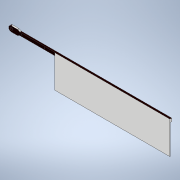
# Autodesk Inventor part: wachlarz_1
Saved by Autodesk Inventor 2022 (Build 260153000, 153)
## iProperties
Created: 2022-12-26
Part Number: wachlarz_1
Material: Generic
Document SubType Name: Modeling
Designer: Kamil
Density: 1 g/cm^3
Appearance: Default
Author: Kamil
Autodesk Inventor part; units mm, degrees
ref_plane "YZ Plane" through (0, 0, 0) normal (1, 0, 0) x (0, 1, 0)
ref_plane "XZ Plane" through (0, 0, 0) normal (0, 1, 0) x (-1, 0, 0)
ref_plane "XY Plane" through (0, 0, 0) normal (0, 0, 1) x (1, 0, 0)
sketch "Sketch1" plane through (0, 0, 0) normal (0, 0, 1) x (1, 0, 0)
  circle A0 centre (0, 3.75) radius 1.75 projected
  line L0 (3.5, -3.25) -> (11.1738, -3.25) projected
  line L1 (11.1738, -3.25) -> (11.1738, -5.25) projected
  line L2 (11.1738, -5.25) -> (-11.1738, -5.25) projected
  line L3 (-11.1738, -5.25) -> (-11.1738, -3.25) projected
  line L4 (-11.1738, -3.25) -> (-3.5, -3.25) projected
  line L5 (-3.5, -3.25) -> (-3.5, 3.75) projected
  arc A1 (3.5, 3.75) -> (-3.5, 3.75) centre (0, 3.75) ccw projected
  line L6 (3.5, 3.75) -> (3.5, -3.25) projected
  line L7 (44, 1.75) -> (50, 1.75) projected
  circle A2 centre (0, 3.75) radius 3.5
  line L8 (0, 3.75) -> (250, 3.75)
  line L9 (50, 1.75) -> (0, 1.75)
  line L10 (0, 1.75) -> (0, 3.75)
  line L11 (0, 3.75) -> (50, 3.75)
  line L12 (50, 3.75) -> (50, 1.75)
  line L13 (50, 1.75) -> (250, 1.75)
  line L14 (250, 1.75) -> (250, 3.75)
  line L15 (250, 3.75) -> (50, 3.75)
  line L16 (50, 3.75) -> (50, 1.75)
  line L17 (0, 1.75) -> (250, 1.75)
  line L18 (250, 1.75) -> (250, 5.75)
  line L19 (250, 5.75) -> (0, 5.75)
  line L20 (0, 5.75) -> (0, 1.75)
  circle A3 centre (0, 3.75) radius 3.5
  point P0 (0, 0)
  point P1 (2.8723, 1.75)
  point P2 (2.8723, 5.75)
  dimension "d0" = 250
  dimension "d1" = 2
  constraints: 26 end point, 6 parallel, 4 horizontal, 3 perpendicular, 2 centre point, 2 coincident, 2 concentric, 1 point on line
  measures "d0" distance of L8.start L8.end
  measures "d1" distance between parallel lines of L8 L19
extrude "Extrusion1" add sketch "Sketch1" along normal blind 2 contours L8 A2 L9 L10 A0 | A0 L20 L19 A1 L8 | A0 L10 L9 A2 A1 L19 L20 | L8 L12 L7 L9 L6 | L6 L9 A2 | A1 L19 L18 L8 | L8 L14 L13 L12
sketch "Sketch2" plane through (0, 0, 2) normal (0, 0, 1) x (1, 0, 0)
  line L0 (13, -15.35) -> (13, -12.35) projected
  line L1 (13, -12.35) -> (14.6, -12.35) projected
  line L2 (14.6, -12.35) -> (14.6, -15.35) projected
  line L3 (14.6, -15.35) -> (13, -15.35) projected
  line L4 (15, -16.35) -> (12.5, -16.35) projected
  line L5 (15, -8.75) -> (15, -16.35) projected
  line L6 (15, -8.75) -> (15, -5.25) projected
  line L7 (12.5, -5.25) -> (15, -5.25) projected
  line L8 (12.5, -16.35) -> (12.5, -5.25) projected
  line L9 (44, -8.25) -> (41.5181, -8.25) projected
  line L10 (44, -9.25) -> (46.5, -9.25) projected
  line L11 (13.75, -5.25) -> (13.75, 7.3756)
  line L12 (44, -8.25) -> (44, 8.5683)
  line L13 (2.8723, 1.75) -> (250, 1.75) projected
  line L14 (250, 1.75) -> (250, 5.75) projected
  line L15 (250, 5.75) -> (2.8723, 5.75) projected
  arc A0 (2.8723, 5.75) -> (2.8723, 1.75) centre (0, 3.75) ccw projected
  circle A1 centre (0, 3.75) radius 1.75 projected
  line L16 (250, 5.75) -> (2.8723, 5.75) projected
  line L17 (13.75, 5.75) -> (13.75, 1.75)
  circle A2 centre (13.75, 3.75) radius 0.5
  line L18 (44, 5.75) -> (44, 1.75)
  line L19 (2.8723, 1.75) -> (250, 1.75) projected
  circle A3 centre (44, 3.75) radius 0.5
  point P0 (0, 0)
  dimension "d4" = 1
  dimension "d5" = 1
  constraints: 8 end point, 8 point on line, 3 midpoint, 2 centre point, 2 vertical
  measures "d4" diameter of A2
  measures "d5" diameter of A3
extrude "Extrusion2" cut sketch "Sketch2" against normal blind 2 contours A2 L11 | L11 A2 | A3 L12 | L12 A3
sketch "Sketch3" plane through (0, 0, 2) normal (0, 0, 1) x (1, 0, 0)
  line L0 (50, -24.1664) -> (50, 13.5237) projected
  circle A0 centre (44, 3.75) radius 0.5 projected
  circle A1 centre (13.75, 3.75) radius 0.5 projected
  line L1 (2.8723, 1.75) -> (250, 1.75) projected
  line L2 (250, 1.75) -> (250, 5.75) projected
  line L3 (250, 5.75) -> (2.8723, 5.75) projected
  arc A2 (2.8723, 5.75) -> (2.8723, 1.75) centre (0, 3.75) ccw projected
  circle A3 centre (0, 3.75) radius 1.75 projected
  line L4 (-50, -43.45) -> (50, -43.45) projected
  line L5 (250, 5.75) -> (57.9443, 5.75)
  line L6 (57.9443, 5.75) -> (57.9443, -37.1171)
  line L7 (57.9443, -37.1171) -> (250, -37.1171)
  line L8 (250, -37.1171) -> (250, 5.75)
  point P0 (0, 0)
  point P1 (57.9443, 5.75)
  constraints: 8 end point, 2 parallel, 1 horizontal, 1 perpendicular
extrude "Extrusion3" add sketch "Sketch3" along normal blind 0.5 contours L6 L3 L2 L1 | L1 L8 L7 L6
sketch "Sketch4" plane through (0, 0, 2.5) normal (0, 0, 1) x (1, 0, 0)
  line L0 (250, -37.1171) -> (250, 5.75) projected
  line L1 (250, 5.75) -> (57.9443, 5.75) projected
  line L2 (57.9443, 5.75) -> (57.9443, -37.1171) projected
  line L3 (57.9443, -37.1171) -> (250, -37.1171) projected
  line L4 (250, -37.1171) -> (250, 1.75) projected
  line L5 (250, -37.1171) -> (210, -37.1171)
  line L6 (210, -37.1171) -> (210, 5.75)
  line L7 (210, 5.75) -> (250, 5.75)
  line L8 (250, 5.75) -> (250, -37.1171)
  point P0 (0, 0)
  dimension "d10" = 40
  constraints: 8 end point, 2 parallel, 1 horizontal, 1 perpendicular, 1 point on line
  measures "d10" distance of L6.end L7.end
extrude "Extrusion4" cut sketch "Sketch4" against normal through all contours L3 L6 L1 L0
sketch "Sketch5" plane through (0, 0, 2) normal (0, 0, 1) x (1, 0, 0)
  line L0 (57.9443, 1.75) -> (57.9443, 5.75) projected
  line L1 (57.9443, 5.75) -> (2.8723, 5.75) projected
  arc A0 (2.8723, 5.75) -> (2.8723, 1.75) centre (0, 3.75) ccw projected
  line L2 (2.8723, 1.75) -> (57.9443, 1.75) projected
  circle A1 centre (44, 3.75) radius 0.5 projected
  circle A2 centre (13.75, 3.75) radius 0.5 projected
  circle A3 centre (0, 3.75) radius 1.75 projected
  arc A4 (2.8723, 5.75) -> (2.8723, 1.75) centre (0, 3.75) ccw projected
  line L3 (0, 0.25) -> (7.7599, 0.25)
  line L4 (8.6265, 0.4475) -> (11.3354, 1.75)
  line L5 (2.8723, 1.75) -> (57.9443, 1.75) projected
  arc A5 (7.7599, 0.25) -> (8.6265, 0.4475) centre (7.7599, 2.25) ccw
  line L6 (0, 3.75) -> (10.3738, 3.75)
  line L7 (0, 7.25) -> (7.7599, 7.25)
  line L8 (8.6265, 7.0525) -> (11.3354, 5.75)
  arc A6 (8.6265, 7.0525) -> (7.7599, 7.25) centre (7.7599, 5.25) ccw
  point P0 (0, 0)
  dimension "d13" = 2
  constraints: 10 end point, 5 point on circle, 5 symmetric about line, 3 tangent, 2 centre point, 2 horizontal, 1 point on line, 1 other
  measures "d13" radius of A5
extrude "Extrusion5" add sketch "Sketch5" against normal up to surface (2 mm away) contours L4 A5 L3 A0 L2 | L1 A0 L7 A6 L8
body "Solid1"
